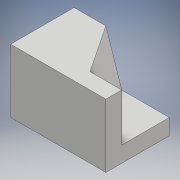
# Autodesk Inventor part: 49
Saved by Autodesk Inventor 2017 (Build 210142000, 142)
## iProperties
Part Number: 49
Material: 一般
Document SubType Name: Modeling
Designer: Brian
Density: 1 g/cm^3
Appearance: 預設
Author: Brian
Autodesk Inventor part; units mm, degrees
ref_plane "YZ Plane" through (0, 0, 0) normal (1, 0, 0) x (0, 1, 0)
ref_plane "XZ Plane" through (0, 0, 0) normal (0, 1, 0) x (-1, 0, 0)
sketch "草圖1" plane through (0, 0, 0) normal (0, 1, 0) x (-1, 0, 0)
  line L0 (0, 0) -> (-60, 0)
  line L1 (-60, 0) -> (-60, -40)
  line L2 (-60, -40) -> (0, -40)
  line L3 (0, -40) -> (0, 0)
  dimension "d0" = 40
  dimension "d1" = 60
  constraints: 8 end point, 2 parallel, 1 horizontal, 1 perpendicular
  measures "d0" distance of L2.end L0.start
  measures "d1" distance of L1.end L2.end
extrude "擠出1" add sketch "草圖1" along normal blind 10
sketch "草圖2" plane through (0, 10, 0) normal (0, 1, 0) x (1, 0, 0)
  line L0 (0, 0) -> (60, 0) projected
  line L1 (20, 0) -> (30, 30)
  line L2 (30, 30) -> (60, 30)
  line L3 (60, 0) -> (60, 40) projected
  line L4 (60, 30) -> (60, 40)
  line L5 (60, 40) -> (0, 40) projected
  line L6 (60, 40) -> (0, 40)
  line L7 (0, 40) -> (0, 0)
  line L8 (20, 0) -> (0, 0)
  dimension "d4" = 10
  dimension "d5" = 30
  dimension "d6" = 30
  constraints: 12 end point, 3 perpendicular, 1 collinear, 1 parallel, 1 point on line
  measures "d4" horizontal distance of L1.start L1.end
  measures "d5" vertical distance of L1.start L1.end
  measures "d6" distance of L1.end L2.end
extrude "擠出2" add sketch "草圖2" along normal blind 30 contours L7 L5 L3 L2 L1 L0
sketch "草圖3" plane through (0, 10, 0) normal (0, 1, 0) x (1, 0, 0)
  line L0 (0, 0) -> (60, 0) projected
  line L1 (40, 0) -> (50, 30)
  line L2 (30, 30) -> (60, 30) projected
  dimension "d9" = 10
  dimension "d10" = 20
  constraints: 2 end point, 2 point on line
  measures "d9" horizontal distance of L1.start L1.end
  measures "d10" distance of L0.end L1.start
ref_plane "工作平面1" through (20, 40, 0) normal (-0.8018, -0.5345, -0.2673) x (0.3162, 0, -0.9487)
sketch "草圖4" plane through (20, 40, 0) normal (-0.8018, -0.5345, -0.2673) x (0.3162, 0, -0.9487)
  line L0 (31.6228, 25.3546) -> (0, 25.3546) projected
  line L1 (31.6228, 25.3546) -> (31.6228, 0) projected
  line L2 (0, 0) -> (31.6228, 0) projected
  line L3 (0, 25.3546) -> (0, 0) projected
  line L4 (41.1096, 40.5674) -> (31.6228, 25.3546) projected
  line L5 (31.6228, 25.3546) -> (0, 25.3546) projected
  line L6 (0, 25.3546) -> (12.6491, 45.6383) projected
  line L7 (12.6491, 45.6383) -> (41.1096, 40.5674) projected
  line L8 (6.3246, 35.4965) -> (37.9473, 35.4965) projected
  line L9 (37.9473, 35.4965) -> (31.6228, 0)
  line L10 (31.6228, 0) -> (41.1096, 15.2128) projected
  line L11 (31.6228, 0) -> (31.6228, 25.3546)
  line L12 (37.9473, 35.4965) -> (31.6228, 25.3546)
  point P0 (-6.3246, 23.6643)
  constraints: 6 end point, 1 collinear, 1 vertical
extrude "擠出3" add sketch "草圖4" along normal up to next contours L1 L2 L3 L0 | L4 L9 L1 | L0 L6 L8 L4
sketch "草圖5" plane through (0, 0, 0) normal (0, 0, 1) x (1, 0, 0)
  line L0 (-0.672, 48.4854) -> (66.1118, 48.4854)
  line L1 (66.1118, 48.4854) -> (66.1118, -3.1014)
  line L2 (66.1118, -3.1014) -> (-0.672, -3.1014)
  line L3 (-0.672, -3.1014) -> (-0.672, 48.4854)
  point P0 (0, 0)
  constraints: 8 end point, 2 parallel, 1 horizontal, 1 perpendicular
extrude "擠出4" cut sketch "草圖5" along normal blind 30
